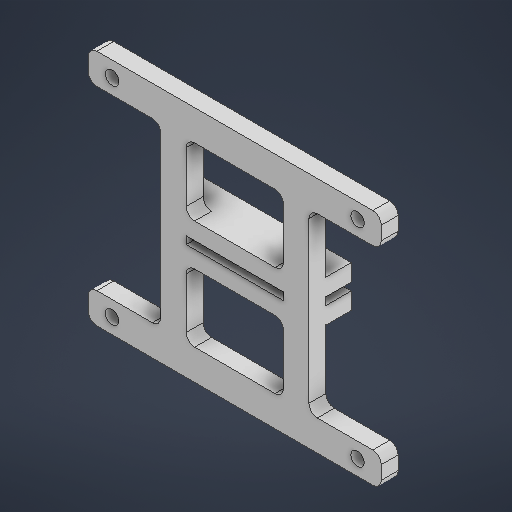
# Autodesk Inventor part: rpi-mount
Saved by Autodesk Inventor 2025 (Build 290162000, 162)
## iProperties
Created: 2024-09-27
Part Number: rpi-mount
Material: Generic
Document SubType Name: Modeling
Designer: Windows 7 was better
Density: 1 g/cm^3
Appearance: Default
Author: Windows 7 was better
Autodesk Inventor part; units mm, degrees
ref_plane "YZ Plane" through (0, 0, 0) normal (1, 0, 0) x (0, 1, 0)
ref_plane "XZ Plane" through (0, 0, 0) normal (0, 1, 0) x (-1, 0, 0)
ref_plane "XY Plane" through (0, 0, 0) normal (0, 0, 1) x (1, 0, 0)
sketch "Sketch1" plane through (0, 0, 0) normal (0, 0, 1) x (1, 0, 0)
  line L0 (0, 0) -> (35, 0)
  line L1 (35, 0) -> (35, -4)
  line L2 (35, -4) -> (0, -4)
  line L3 (0, -4) -> (0, 0)
  line L4 (0, 0) -> (0, 1.8) construction
  line L5 (0, 1.8) -> (35, 1.8)
  line L6 (35, 1.8) -> (35, 5.8)
  line L7 (35, 5.8) -> (0, 5.8)
  line L8 (0, 5.8) -> (0, 1.8)
  line L9 (17.5, 0.9) -> (-11.5, 0.9) construction
  line L10 (-11.5, 0.9) -> (46.5, 0.9) construction
  line L11 (-11.5, 0.9) -> (-11.5, 25.4) construction
  line L12 (-11.5, 25.4) -> (-11.5, -23.6) construction
  line L13 (-11.5, -23.6) -> (46.5, -23.6) construction
  line L14 (-11.5, 25.4) -> (46.5, 25.4) construction
  circle A0 centre (46.5, 25.4) radius 1.6
  circle A1 centre (-11.5, 25.4) radius 1.6
  circle A2 centre (-11.5, -23.6) radius 1.6
  circle A3 centre (46.5, -23.6) radius 1.6
  line L15 (-17.1, -20) -> (52.1, -20)
  line L16 (52.1, -20) -> (52.1, -27.2)
  line L17 (52.1, -27.2) -> (-17.1, -27.2)
  line L18 (-17.1, -27.2) -> (-17.1, -20)
  line L19 (-17.1, -20) -> (52.1, -27.2) construction
  line L20 (52.1, -20) -> (-17.1, -27.2) construction
  line L21 (-17.1, 29) -> (52.1, 29)
  line L22 (52.1, 29) -> (52.1, 21.8)
  line L23 (52.1, 21.8) -> (-17.1, 21.8)
  line L24 (-17.1, 21.8) -> (-17.1, 29)
  line L25 (-17.1, 29) -> (52.1, 21.8) construction
  line L26 (52.1, 29) -> (-17.1, 21.8) construction
  line L27 (35, 21.8) -> (29, 21.8)
  line L28 (29, 21.8) -> (29, -20)
  line L29 (29, -20) -> (35, -20)
  line L30 (35, -20) -> (35, 21.8)
  line L31 (0, 21.8) -> (6, 21.8)
  line L32 (6, 21.8) -> (6, -20)
  line L33 (6, -20) -> (0, -20)
  line L34 (0, -20) -> (0, 21.8)
  point P0 (17.5, -23.6)
  point P1 (17.5, 25.4)
  point P2 (29, 5.8)
  point P3 (6, 5.8)
  point P4 (6, 21.8)
  point P5 (29, 21.8)
  point P6 (29, 0)
  point P7 (6, 0)
  point P8 (6, 1.8)
  point P9 (29, 1.8)
  point P10 (29, -4)
  point P11 (6, -4)
  point P12 (0, -20)
  point P13 (35, -20)
  dimension "d0" = 35
  dimension "d1" = 4
  dimension "d2" = 1.8
  dimension "d3" = 35
  dimension "d4" = 4
  dimension "d5" = 29
  dimension "d6" = 58
  dimension "d7" = 24.5
  dimension "d8" = 49
  dimension "d9" = 58
  dimension "d10" = 58
  dimension "d11" = 3.2
  dimension "d12" = 3.2
  dimension "d13" = 3.2
  dimension "d14" = 3.2
  dimension "d15" = 69.2
  dimension "d16" = 7.2
  dimension "d17" = 69.2
  dimension "d18" = 7.2
  dimension "d19" = 6
  dimension "d20" = 6
  constraints: 70 end point, 12 parallel, 9 horizontal, 6 midpoint, 6 perpendicular, 6 point on line, 4 centre point, 4 coincident, 2 vertical
  measures "d0" distance of L1.end L2.end
  measures "d1" distance of L0.end L1.end
  measures "d2" distance of L0.start L4.end
  measures "d3" distance of L7.end L6.end
  measures "d4" distance of L6.end L5.end
  measures "d5" distance of L9.start L9.end
  measures "d6" distance of L9.end L10.end
  measures "d7" distance of L9.end L11.end
  measures "d8" distance of L11.end L12.end
  measures "d9" distance of L12.end L13.end
  measures "d10" distance of L11.end L14.end
  measures "d11" diameter of A0
  measures "d12" diameter of A1
  measures "d13" diameter of A2
  measures "d14" diameter of A3
  measures "d15" distance of L16.end L17.end
  measures "d16" distance of L15.end L16.end
  measures "d17" distance of L22.end L23.end
  measures "d18" distance of L21.end L22.end
  measures "d19" distance of L29.end L28.end
  measures "d20" distance of L32.end L33.end
extrude "Extrusion1" add sketch "Sketch1" along normal blind 4 contours L34 L5 L32 L0 | L0 L32 L2 L3 | L0 L28 L2 L32 | L2 L32 L15 L34 | L8 L7 L32 L5 | L28 L5 L30 L0 | L0 L1 L2 L28 | L32 L7 L28 L5 | L15 L16 L17 L18 | L34 L23 L32 L7 | L28 L7 L6 L5 | L2 L30 L15 L28 | L23 L24 L21 L22 | L28 L23 L30 L7
extrude "Extrusion2" add sketch "Sketch1" against normal blind 6 contours L0 L32 L2 L3 | L0 L28 L2 L32 | L8 L7 L32 L5 | L0 L1 L2 L28 | L32 L7 L28 L5 | L28 L7 L6 L5
fillet "Fillet1" radius 2 20 edges at (52.1, -27.2, 2) (52.1, -20, 2) (35, -20, 2) (35, 21.8, 2) (52.1, 21.8, 2) (52.1, 29, 2) (-17.1, 29, 2) (-17.1, 21.8, 2) (6, 21.8, 2) (29, 21.8, 2) (0, 21.8, 2) (6, -4, 2) (29, -4, 2) (29, -20, 2) (6, -20, 2) (0, -20, 2) (-17.1, -20, 2) (-17.1, -27.2, 2) (6, 5.8, 2) (29, 5.8, 2)
body "Solid1"
